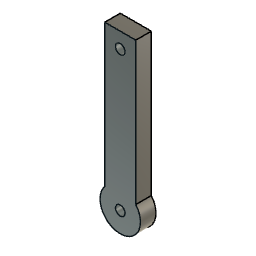
link v3 (Autodesk Fusion 360 design; units mm, degrees)
Autodesk Fusion 360 part; units mm, degrees
sketch "Sketch1" plane through (0, 0, 0) normal (0, 1, 0) x (1, 0, 0)
  line L0 (0, 0) -> (10, 0)
  line L1 (10, 0) -> (10, 45.8467)
  line L2 (0, 45.8467) -> (0, 0)
  line L3 (0, 0) -> (5, 0)
  circle A0 centre (5, 5) radius 1.55
  circle A1 centre (5, 50) radius 1.55
  arc A2 (10, 45.8467) -> (0, 45.8467) centre (5, 50) ccw
  dimension "d1" = 10
  dimension "d4" = 3.1
  dimension "d5" = 3.1
  dimension "d6" = 13
  constraint horizontal L0
  constraint vertical L1
  constraint vertical L2
  constraint coincident L0.start L2.end
  constraint midpoint L0 L3.end
  constraint concentric A1 A2
  measures "d1" distance of L0.start L0.end
  measures "d4" diameter of A0
  measures "d5" diameter of A1
  measures "d6" diameter of A2
extrude "Extrude1" add sketch "Sketch1" along normal blind 5 contours L0 L1 L2 L3 A2 | A0
extrude "Extrude2" add sketch "Sketch1" along normal blind 10 contours L0 L1 L2 L3 A2 | A0
extrude "Extrude3" add sketch "Sketch1" against normal blind 3 contours L0 L1 L2 L3 A2 | A0
extrude "Extrude4" cut 1 faces at (6.6667, 10, -15.2822) along direction (0, -1, 0) blind 2
extrude "Extrude5" add sketch "Sketch1" against normal blind 8 contours A0
delete_face "DeleteFace1" 1 faces at (6.5423, -4.6667, -4.8457)
sketch "Sketch2" plane through (0, 0, 0) normal (0, 1, 0) x (1, 0, 0)
extrude "Extrude7" cut 1 faces at (6.6667, -3, -15.2822) along direction (0, 1, 0) blind 3
extrude "Extrude8" cut sketch "Sketch1" along normal blind 100 contours A0
extrude "Extrude9" cut 1 faces at (5.0386, 0, -32.7463) along direction (0, 1, 0) blind 3
sketch "Sketch3" plane through (0, 3, 0) normal (0, -1, 0) x (1, 0, 0)
  circle A0 centre (5, -5) radius 1.55
  circle A1 centre (5, -50) radius 1.55
  arc A2 (0, -45.8467) -> (10, -45.8467) centre (5, -50) ccw
  line L0 (10, -45.8467) -> (10, 0)
  line L1 (10, 0) -> (0, 0)
  line L2 (0, 0) -> (0, -45.8467)
extrude "Extrude6" [suppressed]
component "Component" placed x (1, 0, 0) y (0, 1, 0) z (0, 0, 1) at (0, 0, 0)
